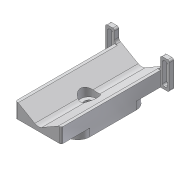
# Autodesk Inventor part: J002880
Saved by Autodesk Inventor 2012 SP2 (Build 160219200, 219)
## iProperties
Created: 2014-07-29
Material: ALUMINUM, 6061-T651
Vendor: HHMI: JFRC - ID&F
Document SubType Name: Modeling
Designer: arnoldj
Density: 2.7 g/cm^3
Part Number: J002880
Description: MPS TUBE HOLDER
Project: P-194005
Mass: 135.792 g
Surface Area: 141.885 cm^2
Volume: 50.2934 cm^3
RuleStatus: InUse
AfterDocSave0: file://Part Number Cleaner
LAB/DEPT: SVOBODA (LAB)
REQUESTING SCIENTIST: PERON, SIMON
SURFACE ROUGHNESS: 63 Ra
DESIGN DEPARTMENT: HHMI: JFRC - ID&F
SPECIAL FINISH: ANODIZE PER MIL-A-8625F, TYPE II, CLASS 2 (BLACK)
ALTERED ITEM PART NUMBER: N/A
ALTERED ITEM VENDOR: N/A
ALTERED ITEM DESCRIPTION: N/A
Revision Number: -
Autodesk Inventor part; units mm, degrees
ref_plane "XY Plane" through (0, 0, 0) normal (0, 0, 1) x (1, 0, 0)
sketch "Sketch1" plane through (0, 0, 0) normal (0, 0, 1) x (1, 0, 0)
  line L0 (-20.701, 0) -> (20.701, 0)
  line L1 (20.701, 0) -> (20.701, 20.193)
  line L2 (-20.701, 20.193) -> (-20.701, 0)
  line L3 (0, 77.3246) -> (0, -12.8874) projected
  line L4 (-35.56, 0) -> (35.56, 0) projected
  line L5 (-18.161, 20.193) -> (0, 9.7077)
  line L6 (0, 9.7077) -> (18.161, 20.193)
  line L7 (20.701, 20.193) -> (18.161, 20.193)
  line L8 (-18.161, 20.193) -> (-20.701, 20.193)
  circle A0 centre (0, 31.6168) radius 18.9738 construction
  circle A1 centre (0, 39.0371) radius 25.4 construction
  point P0 (0, 0)
  point P1 (0, 18.8146)
  dimension "d0" = 41.402
  dimension "d1" = 20.193
  dimension "d2" = 60
  dimension "d3" = 120
  dimension "d4" = 37.9476
  dimension "d5" = 50.8
  dimension "d36" = 2.54
  dimension "d38" = 9.7077
  constraints: 14 end point, 3 parallel, 3 point on line, 2 centre point, 2 tangent, 1 collinear, 1 horizontal, 1 horizontal alignment, 1 perpendicular, 1 vertical alignment, 1 other
  measures "d0" distance of L1.end L2.start
  measures "d1" distance of L2.start L0.start
  measures "d2" angle of L3 L5
  measures "d3" angle of L6 L5
  measures "d4" diameter of A0
  measures "d5" diameter of A1
  measures "d36" distance of L5.start L2.start
  measures "d38" distance from line of L5.end L0
extrude "Extrusion1" add sketch "Sketch1" along normal blind 93.345
sketch "Sketch2" plane through (0, 0, 0) normal (0, 1, 0) x (-1, 0, 0)
  circle A0 centre (0, 46.6725) radius 1.27
  line L0 (18.161, 0) -> (18.161, 93.345) projected
  line L1 (19.05, 14.9225) -> (-19.05, 14.9225)
  line L2 (-19.05, 14.9225) -> (-19.05, 78.4225)
  line L3 (-19.05, 78.4225) -> (19.05, 78.4225)
  line L4 (19.05, 78.4225) -> (19.05, 14.9225)
  point P0 (0, 0)
  point P1 (18.161, 46.6725)
  point P2 (-19.05, 46.6725)
  point P3 (18.161, 46.6725)
  point P4 (0, 78.4225)
  dimension "d8" = 2.54
  dimension "d10" = 38.1
  dimension "d11" = 63.5
  constraints: 8 end point, 4 midpoint, 2 horizontal alignment, 2 parallel, 2 vertical alignment, 1 centre point, 1 horizontal, 1 perpendicular
  measures "d8" diameter of A0
  measures "d10" distance of L2.end L3.end
  measures "d11" distance of L1.end L2.end
ref_plane "Work Plane1 top of part" through (0, 25.4, 0) normal (0, 1, 0) x (-1, 0, 0)
sketch "Sketch3" plane through (0, 25.4, 0) normal (0, 1, 0) x (-1, 0, 0)
  line L0 (-12.7, 78.4225) -> (12.7, 78.4225)
  line L1 (12.7, 78.4225) -> (12.7, 14.9225)
  line L2 (12.7, 14.9225) -> (-12.7, 14.9225)
  line L3 (-12.7, 14.9225) -> (-12.7, 78.4225)
  line L4 (20.701, 0) -> (20.701, 93.345) projected
  line L5 (18.161, 0) -> (18.161, 93.345) projected
  circle A0 centre (0, 46.6725) radius 1.27
  point P0 (0, 0)
  point P1 (0, 78.4225)
  point P2 (12.7, 46.6725)
  point P3 (18.161, 46.6725)
  dimension "d13" = 25.4
  dimension "d14" = 63.5
  dimension "d15" = 2.54
  constraints: 8 end point, 3 midpoint, 2 horizontal alignment, 2 parallel, 1 centre point, 1 horizontal, 1 perpendicular, 1 vertical alignment
  measures "d13" distance of L0.start L0.end
  measures "d14" distance of L2.end L0.start
  measures "d15" diameter of A0
hole "Hole1" [suppressed]
sketch "Sketch4" plane through (0, 25.4, 0) normal (0, 1, 0) x (-1, 0, 0)
  circle A0 centre (0, 47.625) radius 1.27
  line L0 (-20.701, 0) -> (-20.701, 93.345) construction
  line L1 (20.701, 0) -> (20.701, 93.345) projected
  line L2 (-20.701, 46.6725) -> (20.701, 46.6725) construction
  point P0 (0, 0)
  point P1 (0, 46.6725)
  dimension "d60" = 0.9525
  constraints: 3 midpoint, 2 end point, 1 centre point, 1 vertical alignment
  measures "d60" distance from line of L2 A0.centre
hole "Hole2" at (0, 25.4, 47.625) direction (0, -1, 0) diameter 8.255 end through all counterbore diameter 15 counterbore depth 19.685
sketch "Sketch5" plane through (-20.701, 0, 0) normal (0, -1, 0) x (1, 0, 0)
  line L0 (41.402, 93.345) -> (0, 93.345) projected
  line L1 (0, 0) -> (0, 93.345) projected
  line L2 (0, 0) -> (41.402, 0) projected
  line L3 (41.402, 0) -> (41.402, 93.345) projected
  line L4 (0, 78.4225) -> (41.402, 78.4225)
  line L5 (41.402, 78.4225) -> (41.402, 14.9225)
  line L6 (41.402, 14.9225) -> (0, 14.9225)
  line L7 (0, 14.9225) -> (0, 78.4225)
  point P0 (20.701, 0)
  point P1 (0, 46.6725)
  point P2 (0, 46.6725)
  dimension "d39" = 63.5
  constraints: 8 end point, 2 midpoint, 2 parallel, 2 point on line, 1 coincident, 1 horizontal, 1 perpendicular
  measures "d39" distance of L4.end L5.end
extrude "Extrusion2" cut sketch "Sketch5" against normal blind 6.985 contours L3 L4 L1 L0 | L3 L2 L1 L6
fillet "Fillet2" radius 10.795 4 edges at (-20.701, 3.4925, 78.4225) (20.701, 3.4925, 78.4225) (20.701, 3.4925, 14.9225) (-20.701, 3.4925, 14.9225)
fillet "Fillet4" radius 6.35 2 edges at (0, 9.7077, 74.235) (0, 9.7077, 20.0625)
ref_plane "Work Plane2" through (20.701, 0, 0) normal (1, 0, 0) x (0, 1, 0)
ref_plane "Work Plane3" through (-20.701, 0, 0) normal (1, 0, 0) x (0, 1, 0)
sketch "Sketch6" plane through (20.701, 0, 0) normal (1, 0, 0) x (0, 1, 0)
  line L0 (0, 25.7175) -> (0, 67.6275) construction
  line L1 (20.193, 0) -> (20.193, 93.345) construction
  line L2 (0, 46.6725) -> (20.193, 45.72) construction
  point P0 (0, 0)
  point P1 (13.97, 71.4418)
  point P2 (11.5764, 20.6982)
  point P3 (20.32, 1.27)
  point P4 (20.32, 90.17)
  dimension "d47" = 50.8
  dimension "d48" = 13.97
  dimension "d49" = 25.4
  constraints: 2 end point, 1 midpoint, 2 other
  measures "d47" distance of point (11.576, 20.698) point (13.97, 71.442)
  measures "d48" horizontal distance of point (0, 0) point (13.97, 71.442)
  measures "d49" distance from line of L2 point (13.97, 71.442)
hole "Hole3" at (0, 0, 47.625) direction (0, 1, 0) diameter 15 depth 2.794
sketch "Sketch7" plane through (0, 0, 0) normal (0, 0, -1) x (-1, 0, 0)
  line L0 (-20.701, 6.985) -> (-28.829, 6.985)
  line L1 (-28.829, 6.985) -> (-28.829, 31.75)
  line L2 (-28.829, 31.75) -> (-20.701, 31.75)
  line L3 (-20.701, 31.75) -> (-20.701, 6.985)
  line L4 (-18.161, 20.193) -> (-3.175, 11.5408) projected
  line L5 (-18.161, 20.193) -> (-20.701, 21.6595)
  line L6 (-18.161, 20.193) -> (-20.701, 20.193)
  line L7 (-20.701, 20.193) -> (-18.161, 20.193) projected
  line L8 (-20.701, 21.6595) -> (-20.701, 20.193)
  point P0 (0, 0)
  dimension "d63" = 8.128
  dimension "d64" = 24.765
  constraints: 14 end point, 3 perpendicular, 2 parallel, 1 collinear, 1 horizontal, 1 point on line
  measures "d63" distance of L1.end L2.end
  measures "d64" distance of L0.end L1.end
extrude "Extrusion3" add sketch "Sketch7" against normal blind 3.81
sketch "Sketch8" plane through (0, 0, 0) normal (0, 0, -1) x (-1, 0, 0)
  line L0 (-20.701, 31.75) -> (-28.829, 31.75) projected
  line L1 (-28.829, 31.75) -> (-28.829, 6.985) projected
  line L2 (-26.924, 29.591) -> (-22.606, 29.591)
  line L3 (-22.606, 29.591) -> (-22.606, 9.144)
  line L4 (-22.606, 9.144) -> (-26.924, 9.144)
  line L5 (-26.924, 9.144) -> (-26.924, 29.591)
  line L6 (-24.765, 29.591) -> (-24.765, 9.144) construction
  line L7 (-26.924, 19.3675) -> (-22.606, 19.3675) construction
  point P0 (0, 0)
  point P1 (-24.765, 31.75)
  point P2 (-28.829, 19.3675)
  dimension "d67" = 4.318
  dimension "d68" = 20.447
  constraints: 12 end point, 6 midpoint, 2 parallel, 1 horizontal, 1 horizontal alignment, 1 perpendicular, 1 vertical alignment
  measures "d67" distance of L2.start L2.end
  measures "d68" distance of L4.end L2.start
extrude "Extrusion4" cut sketch "Sketch8" against normal up to next
fillet "Fillet6" radius 1.5875 3 edges at (20.701, 31.75, 1.905) (28.829, 31.75, 1.905) (28.829, 6.985, 1.905)
fillet "Fillet7" radius 1.5875 4 edges at (26.924, 29.591, 1.905) (22.606, 29.591, 1.905) (22.606, 9.144, 1.905) (26.924, 9.144, 1.905)
mirror "Mirror2" about plane through (0, 0, 0) normal (1, 0, 0) of "Extrusion3", "Extrusion4", "Fillet6", "Fillet7"
fillet "Fillet8" radius 3.175 1 edges at (-20.701, 21.6595, 1.905)
fillet "Fillet9" radius 1.5875 2 edges at (20.701, 13.589, 93.345) (-20.701, 13.589, 93.345)
fillet "Fillet10" radius 3.175 1 edges at (20.701, 21.6595, 1.905)
body "Solid1"
